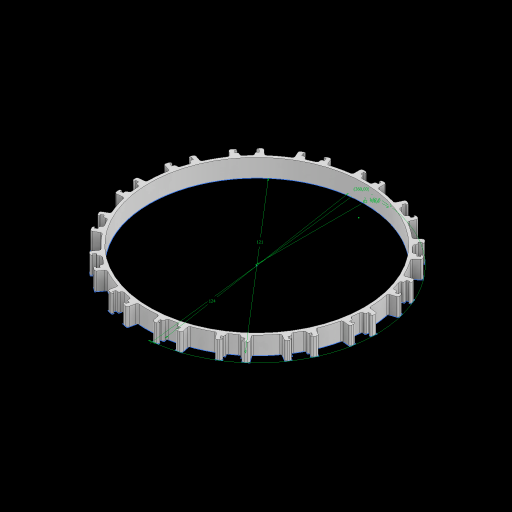
# Autodesk Inventor part: MM-D120
Saved by Autodesk Inventor 2024.2 (Build 282272000, 272)
## iProperties
Created: 2024-10-21
Part Number: MM-D120
Material: Generic
Document SubType Name: Modeling
Designer: Mikonator
Density: 1 g/cm^3
Appearance: Default
Author: Mikonator
Autodesk Inventor part; units mm, degrees
ref_plane "YZ Plane" through (0, 0, 0) normal (1, 0, 0) x (0, 1, 0)
ref_plane "XZ Plane" through (0, 0, 0) normal (0, 1, 0) x (-1, 0, 0)
ref_plane "XY Plane" through (0, 0, 0) normal (0, 0, 1) x (1, 0, 0)
sketch "Sketch1" plane through (0, 0, 0) normal (0, 1, 0) x (-1, 0, 0)
  line L0 (-1, -14.604) -> (1.9819, -14.604)
  line L1 (1.9819, -14.604) -> (1.9819, -13.604)
  line L2 (1.9819, -13.604) -> (0.9819, -13.604)
  line L3 (0.9819, -13.604) -> (0.9819, -12.004)
  line L4 (2.835, -12.004) -> (2.835, -10.004)
  line L5 (2.835, -10.004) -> (6.035, -10.004)
  line L6 (4.5819, -8.4996) -> (4.5819, -8.4996)
  line L7 (13, -14.604) -> (9.7145, -14.604)
  line L8 (9.7145, -14.604) -> (9.7145, -13.604)
  line L9 (9.7145, -13.604) -> (10.7145, -13.604)
  line L10 (10.7145, -13.604) -> (10.7145, -12.004)
  line L11 (10.7145, -12.004) -> (8.9145, -12.004)
  line L12 (8.9145, -12.004) -> (8.9145, -10.004)
  line L13 (8.9145, -10.004) -> (6.035, -10.004)
  circle A0 centre (5.3117, 51.996) radius 62
  line L14 (2.835, -12.004) -> (0.9819, -12.004)
  circle A1 centre (5.3117, 51.996) radius 60.5
  line L15 (13, -14.604) -> (13, -9.5255)
  line L16 (-1, -14.604) -> (-1, -9.6819)
  line L17 (39.424, -5.719) -> (36.4226, -7.0553)
  line L18 (36.4226, -7.0553) -> (36.0158, -6.1418)
  line L19 (36.0158, -6.1418) -> (36.9294, -5.735)
  line L20 (36.9294, -5.735) -> (36.2786, -4.2734)
  line L21 (39.424, -5.719) -> (37.3583, -1.0795)
  line L22 (36.2786, -4.2734) -> (34.6342, -5.0055)
  line L23 (34.6342, -5.0055) -> (33.8207, -3.1784)
  line L24 (33.8207, -3.1784) -> (31.1901, -4.3496)
  line L25 (28.2668, -5.6512) -> (31.1901, -4.3496)
  line L26 (29.0803, -7.4783) -> (28.2668, -5.6512)
  line L27 (29.0803, -7.4783) -> (27.3874, -8.232)
  line L28 (28.0382, -9.6937) -> (27.3874, -8.232)
  line L29 (28.9517, -9.2869) -> (28.0382, -9.6937)
  line L30 (29.3584, -10.2005) -> (28.9517, -9.2869)
  line L31 (26.6343, -11.4133) -> (29.3584, -10.2005)
  line L32 (26.6343, -11.4133) -> (24.6323, -6.9168)
  line L33 (59.9496, 13.1454) -> (57.7512, 10.7039)
  line L34 (57.7512, 10.7039) -> (57.0081, 11.373)
  line L35 (57.0081, 11.373) -> (57.6772, 12.1161)
  line L36 (57.6772, 12.1161) -> (56.4882, 13.1867)
  line L37 (59.9496, 13.1454) -> (56.1755, 16.5436)
  line L38 (56.4882, 13.1867) -> (55.2837, 11.8491)
  line L39 (55.2837, 11.8491) -> (53.7974, 13.1873)
  line L40 (53.7974, 13.1873) -> (51.8707, 11.0474)
  line L41 (49.7294, 8.6694) -> (51.8707, 11.0474)
  line L42 (51.2157, 7.3311) -> (49.7294, 8.6694)
  line L43 (51.2157, 7.3311) -> (49.9758, 5.954)
  line L44 (51.1648, 4.8834) -> (49.9758, 5.954)
  line L45 (51.8339, 5.6265) -> (51.1648, 4.8834)
  line L46 (52.5771, 4.9574) -> (51.8339, 5.6265)
  line L47 (50.5818, 2.7414) -> (52.5771, 4.9574)
  line L48 (50.5818, 2.7414) -> (46.9239, 6.0349)
  line L49 (71.0279, 38.7275) -> (70.0126, 35.6028)
  line L50 (70.0126, 35.6028) -> (69.0615, 35.9119)
  line L51 (69.0615, 35.9119) -> (69.3706, 36.8629)
  line L52 (69.3706, 36.8629) -> (67.8489, 37.3573)
  line L53 (71.0279, 38.7275) -> (66.1979, 40.2968)
  line L54 (67.8489, 37.3573) -> (67.2926, 35.6454)
  line L55 (67.2926, 35.6454) -> (65.3905, 36.2635)
  line L56 (65.3905, 36.2635) -> (64.5007, 33.5249)
  line L57 (63.5118, 30.4815) -> (64.5007, 33.5249)
  line L58 (65.414, 29.8634) -> (63.5118, 30.4815)
  line L59 (65.414, 29.8634) -> (64.8413, 28.1011)
  line L60 (66.363, 27.6066) -> (64.8413, 28.1011)
  line L61 (66.672, 28.5577) -> (66.363, 27.6066)
  line L62 (67.6231, 28.2487) -> (66.672, 28.5577)
  line L63 (66.7016, 25.4127) -> (67.6231, 28.2487)
  line L64 (66.7016, 25.4127) -> (62.0204, 26.9337)
  line L65 (70.7432, 66.6038) -> (71.0866, 63.3363)
  line L66 (71.0866, 63.3363) -> (70.0921, 63.2318)
  line L67 (70.0921, 63.2318) -> (69.9875, 64.2263)
  line L68 (69.9875, 64.2263) -> (68.3963, 64.0591)
  line L69 (70.7432, 66.6038) -> (65.6925, 66.0729)
  line L70 (68.3963, 64.0591) -> (68.5845, 62.269)
  line L71 (68.5845, 62.269) -> (66.5954, 62.0599)
  line L72 (66.5954, 62.0599) -> (66.8964, 59.1961)
  line L73 (67.2309, 56.0137) -> (66.8964, 59.1961)
  line L74 (69.22, 56.2227) -> (67.2309, 56.0137)
  line L75 (69.22, 56.2227) -> (69.4137, 54.3798)
  line L76 (71.0049, 54.547) -> (69.4137, 54.3798)
  line L77 (70.9004, 55.5415) -> (71.0049, 54.547)
  line L78 (71.8949, 55.6461) -> (70.9004, 55.5415)
  line L79 (72.2066, 52.6805) -> (71.8949, 55.6461)
  line L80 (72.2066, 52.6805) -> (67.3114, 52.166)
  line L81 (59.1448, 91.9543) -> (60.7875, 89.109)
  line L82 (60.7875, 89.109) -> (59.9215, 88.609)
  line L83 (59.9215, 88.609) -> (59.4215, 89.475)
  line L84 (59.4215, 89.475) -> (58.0359, 88.675)
  line L85 (59.1448, 91.9543) -> (54.7466, 89.415)
  line L86 (58.0359, 88.675) -> (58.9359, 87.1162)
  line L87 (58.9359, 87.1162) -> (57.2038, 86.1162)
  line L88 (57.2038, 86.1162) -> (58.6436, 83.6224)
  line L89 (60.2436, 80.8511) -> (58.6436, 83.6224)
  line L90 (61.9756, 81.8511) -> (60.2436, 80.8511)
  line L91 (61.9756, 81.8511) -> (62.9022, 80.2463)
  line L92 (64.2878, 81.0463) -> (62.9022, 80.2463)
  line L93 (63.7878, 81.9123) -> (64.2878, 81.0463)
  line L94 (64.6538, 82.4123) -> (63.7878, 81.9123)
  line L95 (66.1448, 79.8299) -> (64.6538, 82.4123)
  line L96 (66.1448, 79.8299) -> (61.8821, 77.3689)
  line L97 (38.2382, 110.3956) -> (40.8962, 108.4645)
  line L98 (40.8962, 108.4645) -> (40.3084, 107.6554)
  line L99 (40.3084, 107.6554) -> (39.4994, 108.2432)
  line L100 (39.4994, 108.2432) -> (38.5589, 106.9488)
  line L101 (38.2382, 110.3956) -> (35.2531, 106.287)
  line L102 (38.5589, 106.9488) -> (40.0151, 105.8908)
  line L103 (40.0151, 105.8908) -> (38.8396, 104.2728)
  line L104 (38.8396, 104.2728) -> (41.1692, 102.5802)
  line L105 (43.758, 100.6993) -> (41.1692, 102.5802)
  line L106 (44.9336, 102.3173) -> (43.758, 100.6993)
  line L107 (44.9336, 102.3173) -> (46.4328, 101.2281)
  line L108 (47.3732, 102.5225) -> (46.4328, 101.2281)
  line L109 (46.5642, 103.1103) -> (47.3732, 102.5225)
  line L110 (47.152, 103.9193) -> (46.5642, 103.1103)
  line L111 (49.5644, 102.1666) -> (47.152, 103.9193)
  line L112 (49.5644, 102.1666) -> (46.6713, 98.1845)
  line L113 (11.6383, 118.7391) -> (14.8519, 118.056)
  line L114 (14.8519, 118.056) -> (14.644, 117.0779)
  line L115 (14.644, 117.0779) -> (13.6659, 117.2858)
  line L116 (13.6659, 117.2858) -> (13.3332, 115.7208)
  line L117 (11.6383, 118.7391) -> (10.5824, 113.7715)
  line L118 (13.3332, 115.7208) -> (15.0939, 115.3465)
  line L119 (15.0939, 115.3465) -> (14.678, 113.3902)
  line L120 (14.678, 113.3902) -> (17.4947, 112.7915)
  line L121 (20.6247, 112.1262) -> (17.4947, 112.7915)
  line L122 (21.0406, 114.0825) -> (20.6247, 112.1262)
  line L123 (21.0406, 114.0825) -> (22.8532, 113.6972)
  line L124 (23.1858, 115.2623) -> (22.8532, 113.6972)
  line L125 (22.2077, 115.4702) -> (23.1858, 115.2623)
  line L126 (22.4156, 116.4483) -> (22.2077, 115.4702)
  line L127 (25.3323, 115.8283) -> (22.4156, 116.4483)
  line L128 (25.3323, 115.8283) -> (24.309, 111.0138)
  line L129 (-16.0556, 115.5421) -> (-12.8419, 116.2252)
  line L130 (-12.8419, 116.2252) -> (-12.634, 115.2471)
  line L131 (-12.634, 115.2471) -> (-13.6122, 115.0391)
  line L132 (-13.6122, 115.0391) -> (-13.2795, 113.4741)
  line L133 (-16.0556, 115.5421) -> (-14.9997, 110.5746)
  line L134 (-13.2795, 113.4741) -> (-11.5188, 113.8483)
  line L135 (-11.5188, 113.8483) -> (-11.103, 111.8921)
  line L136 (-11.103, 111.8921) -> (-8.2864, 112.4907)
  line L137 (-5.1563, 113.1561) -> (-8.2864, 112.4907)
  line L138 (-5.5721, 115.1124) -> (-5.1563, 113.1561)
  line L139 (-5.5721, 115.1124) -> (-3.7595, 115.4976)
  line L140 (-4.0922, 117.0627) -> (-3.7595, 115.4976)
  line L141 (-5.0703, 116.8548) -> (-4.0922, 117.0627)
  line L142 (-5.2783, 117.8329) -> (-5.0703, 116.8548)
  line L143 (-2.3615, 118.4529) -> (-5.2783, 117.8329)
  line L144 (-2.3615, 118.4529) -> (-1.3381, 113.6383)
  line L145 (-40.0548, 101.3574) -> (-37.3968, 103.2886)
  line L146 (-37.3968, 103.2886) -> (-36.8091, 102.4796)
  line L147 (-36.8091, 102.4796) -> (-37.6181, 101.8918)
  line L148 (-37.6181, 101.8918) -> (-36.6776, 100.5973)
  line L149 (-40.0548, 101.3574) -> (-37.0697, 97.2488)
  line L150 (-36.6776, 100.5973) -> (-35.2214, 101.6554)
  line L151 (-35.2214, 101.6554) -> (-34.0458, 100.0373)
  line L152 (-34.0458, 100.0373) -> (-31.7162, 101.7299)
  line L153 (-29.1274, 103.6108) -> (-31.7162, 101.7299)
  line L154 (-30.3029, 105.2288) -> (-29.1274, 103.6108)
  line L155 (-30.3029, 105.2288) -> (-28.8037, 106.318)
  line L156 (-29.7442, 107.6125) -> (-28.8037, 106.318)
  line L157 (-30.5532, 107.0247) -> (-29.7442, 107.6125)
  line L158 (-31.141, 107.8337) -> (-30.5532, 107.0247)
  line L159 (-28.7286, 109.5864) -> (-31.141, 107.8337)
  line L160 (-28.7286, 109.5864) -> (-25.8354, 105.6044)
  line L161 (-56.2098, 78.6377) -> (-54.5671, 81.483)
  line L162 (-54.5671, 81.483) -> (-53.701, 80.983)
  line L163 (-53.701, 80.983) -> (-54.201, 80.117)
  line L164 (-54.201, 80.117) -> (-52.8154, 79.317)
  line L165 (-56.2098, 78.6377) -> (-51.8116, 76.0984)
  line L166 (-52.8154, 79.317) -> (-51.9154, 80.8758)
  line L167 (-51.9154, 80.8758) -> (-50.1833, 79.8758)
  line L168 (-50.1833, 79.8758) -> (-48.7436, 82.3696)
  line L169 (-47.1436, 85.1408) -> (-48.7436, 82.3696)
  line L170 (-48.8756, 86.1408) -> (-47.1436, 85.1408)
  line L171 (-48.8756, 86.1408) -> (-47.9491, 87.7457)
  line L172 (-49.3347, 88.5457) -> (-47.9491, 87.7457)
  line L173 (-49.8347, 87.6796) -> (-49.3347, 88.5457)
  line L174 (-50.7007, 88.1796) -> (-49.8347, 87.6796)
  line L175 (-49.2098, 90.762) -> (-50.7007, 88.1796)
  line L176 (-49.2098, 90.762) -> (-44.9471, 88.301)
  line L177 (-61.7271, 51.3114) -> (-61.3837, 54.5788)
  line L178 (-61.3837, 54.5788) -> (-60.3892, 54.4743)
  line L179 (-60.3892, 54.4743) -> (-60.4937, 53.4798)
  line L180 (-60.4937, 53.4798) -> (-58.9025, 53.3125)
  line L181 (-61.7271, 51.3114) -> (-56.6764, 50.7805)
  line L182 (-58.9025, 53.3125) -> (-58.7143, 55.1027)
  line L183 (-58.7143, 55.1027) -> (-56.7253, 54.8936)
  line L184 (-56.7253, 54.8936) -> (-56.4243, 57.7574)
  line L185 (-56.0898, 60.9398) -> (-56.4243, 57.7574)
  line L186 (-58.0789, 61.1489) -> (-56.0898, 60.9398)
  line L187 (-58.0789, 61.1489) -> (-57.8852, 62.9918)
  line L188 (-59.4764, 63.1591) -> (-57.8852, 62.9918)
  line L189 (-59.5809, 62.1646) -> (-59.4764, 63.1591)
  line L190 (-60.5754, 62.2691) -> (-59.5809, 62.1646)
  line L191 (-60.2637, 65.2347) -> (-60.5754, 62.2691)
  line L192 (-60.2637, 65.2347) -> (-55.3686, 64.7202)
  line L193 (-55.6529, 24.1034) -> (-56.6681, 27.2281)
  line L194 (-56.6681, 27.2281) -> (-55.7171, 27.5371)
  line L195 (-55.7171, 27.5371) -> (-55.4081, 26.586)
  line L196 (-55.4081, 26.586) -> (-53.8864, 27.0805)
  line L197 (-55.6529, 24.1034) -> (-50.8229, 25.6728)
  line L198 (-53.8864, 27.0805) -> (-54.4426, 28.7924)
  line L199 (-54.4426, 28.7924) -> (-52.5405, 29.4104)
  line L200 (-52.5405, 29.4104) -> (-53.4303, 32.149)
  line L201 (-54.4192, 35.1924) -> (-53.4303, 32.149)
  line L202 (-56.3213, 34.5743) -> (-54.4192, 35.1924)
  line L203 (-56.3213, 34.5743) -> (-56.8939, 36.3367)
  line L204 (-58.4156, 35.8423) -> (-56.8939, 36.3367)
  line L205 (-58.1066, 34.8913) -> (-58.4156, 35.8423)
  line L206 (-59.0576, 34.5822) -> (-58.1066, 34.8913)
  line L207 (-59.9791, 37.4182) -> (-59.0576, 34.5822)
  line L208 (-59.9791, 37.4182) -> (-55.2979, 38.9392)
  line L209 (-39.0373, 1.7183) -> (-41.2357, 4.1599)
  line L210 (-41.2357, 4.1599) -> (-40.4925, 4.829)
  line L211 (-40.4925, 4.829) -> (-39.8234, 4.0859)
  line L212 (-39.8234, 4.0859) -> (-38.6344, 5.1565)
  line L213 (-39.0373, 1.7183) -> (-35.2632, 5.1166)
  line L214 (-38.6344, 5.1565) -> (-39.8388, 6.4942)
  line L215 (-39.8388, 6.4942) -> (-38.3525, 7.8324)
  line L216 (-38.3525, 7.8324) -> (-40.2793, 9.9723)
  line L217 (-42.4205, 12.3504) -> (-40.2793, 9.9723)
  line L218 (-43.9068, 11.0121) -> (-42.4205, 12.3504)
  line L219 (-43.9068, 11.0121) -> (-45.1468, 12.3893)
  line L220 (-46.3358, 11.3187) -> (-45.1468, 12.3893)
  line L221 (-45.6667, 10.5755) -> (-46.3358, 11.3187)
  line L222 (-46.4098, 9.9064) -> (-45.6667, 10.5755)
  line L223 (-48.4051, 12.1224) -> (-46.4098, 9.9064)
  line L224 (-48.4051, 12.1224) -> (-44.7473, 15.4159)
  line L225 (-14.7534, -11.9733) -> (-17.7548, -10.637)
  line L226 (-17.7548, -10.637) -> (-17.348, -9.7234)
  line L227 (-17.348, -9.7234) -> (-16.4345, -10.1301)
  line L228 (-16.4345, -10.1301) -> (-15.7837, -8.6685)
  line L229 (-14.7534, -11.9733) -> (-12.6877, -7.3338)
  line L230 (-15.7837, -8.6685) -> (-17.4281, -7.9363)
  line L231 (-17.4281, -7.9363) -> (-16.6146, -6.1093)
  line L232 (-16.6146, -6.1093) -> (-19.2452, -4.938)
  line L233 (-22.1686, -3.6365) -> (-19.2452, -4.938)
  line L234 (-22.982, -5.4636) -> (-22.1686, -3.6365)
  line L235 (-22.982, -5.4636) -> (-24.6749, -4.7099)
  line L236 (-25.3257, -6.1715) -> (-24.6749, -4.7099)
  line L237 (-24.4121, -6.5783) -> (-25.3257, -6.1715)
  line L238 (-24.8189, -7.4918) -> (-24.4121, -6.5783)
  line L239 (-27.543, -6.279) -> (-24.8189, -7.4918)
  line L240 (-27.543, -6.279) -> (-25.541, -1.7824)
  point P0 (0, 0)
  dimension "d16" = 124
  dimension "d34" = 121
  dimension "d4" = 1
  dimension "d5" = 2
  dimension "d8" = 3.6
  dimension "d9" = 2.6
  dimension "d10" = 3.2
  dimension "d12" = 1.6
  dimension "d25" = 62
  dimension "d28" = 360
  constraints: 468 end point, 12 perpendicular, 2 vertical, 1 coincident, 1 horizontal, 503 other
  measures "d4" distance between parallel lines of L0 L2
  measures "d5" distance of L4.start L4.end
  measures "d8" distance between parallel lines of L3 L6
  measures "d9" distance between parallel lines of L1 L6
  measures "d10" distance of L4.end L5.end
  measures "d12" distance of L2.end L3.end
  measures "d25" vertical distance of point (5.312, 51.996) L5.end
extrude "Extrusion3" add sketch "Sketch1" along normal blind 10 contours L16 A0 L5 L4 L14 L3 L2 L1 L0 | A0 | L229 L225 L226 L227 L228 L230 L231 L232 L233 A0 | A0 L15 L7 L8 L9 L10 L11 L12 L13 L5 | L233 L234 L235 L236 L237 L238 L239 L240 A0 | A0 L25 L26 L27 L28 L29 L30 L31 L32 | L213 L209 L210 L211 L212 L214 L215 L216 L217 A0 | A0 L21 L17 L18 L19 L20 L22 L23 L24 L25 | L217 L218 L219 L220 L221 L222 L223 L224 A0 | A0 L41 L42 L43 L44 L45 L46 L47 L48 | L197 L193 L194 L195 L196 L198 L199 L200 L201 A0 | A0 L37 L33 L34 L35 L36 L38 L39 L40 L41 | L201 L202 L203 L204 L205 L206 L207 L208 A0 | A0 L57 L58 L59 L60 L61 L62 L63 L64 | L181 L177 L178 L179 L180 L182 L183 L184 L185 A0 | A0 L53 L49 L50 L51 L52 L54 L55 L56 L57 | L185 L186 L187 L188 L189 L190 L191 L192 A0 | L165 L161 L162 L163 L164 L166 L167 L168 L169 A0 | A0 L73 L74 L75 L76 L77 L78 L79 L80 | L169 L170 L171 L172 L173 L174 L175 L176 A0 | A0 L69 L65 L66 L67 L68 L70 L71 L72 L73 | L149 L145 L146 L147 L148 L150 L151 L152 L153 A0 | A0 L89 L90 L91 L92 L93 L94 L95 L96 | L153 L154 L155 L156 L157 L158 L159 L160 A0 | A0 L85 L81 L82 L83 L84 L86 L87 L88 L89 | L133 L129 L130 L131 L132 L134 L135 L136 L137 A0 | A0 L105 L106 L107 L108 L109 L110 L111 L112 | L137 L138 L139 L140 L141 L142 L143 L144 A0 | A0 L101 L97 L98 L99 L100 L102 L103 L104 L105 | L117 L113 L114 L115 L116 L118 L119 L120 L121 A0 | A0 L121 L122 L123 L124 L125 L126 L127 L128 | A1
extrude "Extrusion4" cut sketch "Sketch1" along normal through all contours A1
fillet "Fillet1" radius 1 10 edges at (1, 5, -9.6819) (1, 5, -14.604) (-1.9819, 5, -14.604) (-9.7145, 5, -14.604) (-13, 5, -14.604) (-2.835, 5, -12.004) (-2.835, 5, -10.004) (-8.9145, 5, -10.004) (-8.9145, 5, -12.004) (-13, 5, -9.5255)
pattern_circular "Circular Pattern1" count 15 over 360 about axis through (-5.3117, 0, 51.996) along (0, 1, 0) of "Fillet1"
body "Solid3"
